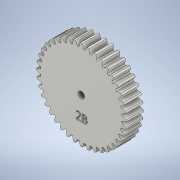
# Autodesk Inventor part: Spur Gear1
Saved by Autodesk Inventor 2021 (Build 250183000, 183)
## iProperties
CustomPartVersion: 1
Created: 2021-04-14
Part Number: Spur Gear1
Material: Steel
Document SubType Name: Modeling
Designer: Nabeel Azafer
Categories: <?xml version="1.0" encoding="UTF-16"?> <MemberInstance><Categories><FamilyTemplate><FamilyTemplateParameter ValueType="xs:double" Id="1" ObjectReferenceKey="da_z" ObjectType="kUserParameterObject"/><FamilyTemplateParameter ValueType="xs:double" Id="2" ObjectReferenceKey="da_b" ObjectType="kUserParameterObject"/><FamilyTemplateParameter ValueType="xs:double" Id="3" ObjectReferenceKey="da_beta" ObjectType="kUserParameterObject"/><FamilyTemplateParameter ValueType="xs:double" Id="4" ObjectReferenceKey="da_da" ObjectType="kUserParameterObject"/><FamilyTemplateParameter ValueType="xs:double" Id="5" ObjectReferenceKey="da_aw" ObjectType="kUserParameterObject"/><FamilyTemplateParameter ValueType="xs:string" Id="6" ObjectReferenceKey="EAIAABAAAACIAQAAAAAAAIAAAAAAAAAA" ObjectType="83910656" SubObjectId="SurfaceGeometry"/></FamilyTemplate><ParamToTemplateMap><ParamToTemplate CategoryParameter="//CategoryParameter[@InternalName='046C89C9-8512-4d59-83FE-43B91F4F132A']" TemplateParameter="1"/><ParamToTemplate CategoryParameter="//CategoryParameter[@InternalName='2552DF32-E462-4b46-AEBF-C6C7768E72AC']" TemplateParameter="2"/><ParamToTemplate CategoryParameter="//CategoryParameter[@InternalName='C9EE641D-15FC-4fae-A226-E94C4372FDD7']" TemplateParameter="3"/><ParamToTemplate><ParamToTemplate CategoryParameter="//CategoryParameter[@InternalName='00B6519A-459B-49c7-AD84-2E56D39A5744']" ConstantValue="0.000000"/></ParamToTemplate><ParamToTemplate><ParamToTemplate CategoryParameter="//CategoryParameter[@InternalName='04B31F0E-C7A6-4894-AA32-9629BEFACF47']" ConstantValue="0.800000"/></ParamToTemplate><ParamToTemplate><ParamToTemplate CategoryParameter="//CategoryParameter[@InternalName='43CBEC2E-7847-49e7-A936-2F7889FCB2D9']" ConstantValue="0.350000"/></ParamToTemplate><ParamToTemplate><ParamToTemplate CategoryParameter="//CategoryParameter[@InternalName='B1EFC894-105D-4ebd-86BF-FA20ED196853']" ConstantValue="0.500000"/></ParamToTemplate><ParamToTemplate><ParamToTemplate CategoryParameter="//CategoryParameter[@InternalName='51175063-3D10-4879-93E8-6246FE8B403D']" ConstantValue="2060000000.000000"/></ParamToTemplate><ParamToTemplate><ParamToTemplate CategoryParameter="//CategoryParameter[@InternalName='A3A52E27-4454-46a9-B0BD-C932399B70AF']" ConstantValue="0.300000"/></ParamToTemplate><ParamToTemplate><ParamToTemplate CategoryParameter="//CategoryParameter[@InternalName='91B76062-C214-41d9-B1B9-14D2AB99603D']" ConstantValue="0.100000"/></ParamToTemplate><ParamToTemplate><ParamToTemplate CategoryParameter="//CategoryParameter[@InternalName='374E806E-8B8A-4dda-A9AA-1039D6500AD2']" ConstantValue="10.000000"/></ParamToTemplate><ParamToTemplate><ParamToTemplate CategoryParameter="//CategoryParameter[@InternalName='2D373A89-B862-43d6-8D0B-0CBF12AB9F6C']" ConstantValue="0.349066"/></ParamToTemplate><ParamToTemplate CategoryParameter="//CategoryParameter[@InternalName='37777632-D6A2-4fac-9D53-DB8ACD95C989']" TemplateParameter="4"/><ParamToTemplate CategoryParameter="//CategoryParameter[@InternalName='FD1017F1-B727-4f7e-9707-0F86F1FF9423']" TemplateParameter="5"/><ParamToTemplate><ParamToTemplate CategoryParameter="//CategoryParameter[@InternalName='9E1B4470-B2D3-4ff1-B813-535BB4CDF51A']" ConstantValue="3520000.000000"/></ParamToTemplate><ParamToTemplate><ParamToTemplate CategoryParameter="//CategoryParameter[@InternalName='F8452263-BFF6-458c-9FB1-07C4B99E95CD']" ConstantValue="11400000.000000"/></ParamToTemplate><ParamToTemplate><ParamToTemplate CategoryParameter="//CategoryParameter[@InternalName='3E3BB259-FD49-497f-8171-6EBC954A3479']" ConstantValue="2.000000"/></ParamToTemplate><ParamToTemplate CategoryParameter="//CategoryParameter[@InternalName='27C3BAF2-7550-4e4b-AE2C-0DB134B7D9B7']" TemplateParameter="6"/></ParamToTemplateMap><Category DisplayName="Gear" InternalName="DC85795E-93AB-48d5-8EEE-5A27447B64BD" Mnemonic="Gear"><CategoryParameter DisplayName="z" InternalName="046C89C9-8512-4d59-83FE-43B91F4F132A" Mnemonic="z"/><CategoryParameter DisplayName="b" InternalName="2552DF32-E462-4b46-AEBF-C6C7768E72AC" Mnemonic="b"/><CategoryParameter DisplayName="||b|" InternalName="C9EE641D-15FC-4fae-A226-E94C4372FDD7" Mnemonic="beta"/><CategoryParameter DisplayName="x" InternalName="00B6519A-459B-49c7-AD84-2E56D39A5744" Mnemonic="x"/><CategoryParameter DisplayName="a*" InternalName="04B31F0E-C7A6-4894-AA32-9629BEFACF47" Mnemonic="a"/><CategoryParameter DisplayName="c*" InternalName="43CBEC2E-7847-49e7-A936-2F7889FCB2D9" Mnemonic="c"/><CategoryParameter DisplayName="r|.f|*" InternalName="B1EFC894-105D-4ebd-86BF-FA20ED196853" Mnemonic="rf"/><CategoryParameter DisplayName="E" InternalName="51175063-3D10-4879-93E8-6246FE8B403D" Mnemonic="E"/><CategoryParameter DisplayName="||m|" InternalName="A3A52E27-4454-46a9-B0BD-C932399B70AF" Mnemonic="mi"/><Category DisplayName="SpurGear" InternalName="26C5A22E-A91E-4dfd-A3B3-23CCAFAE1764" Mnemonic="SpurGear"><CategoryParameter DisplayName="m" InternalName="91B76062-C214-41d9-B1B9-14D2AB99603D" Mnemonic="m"/><CategoryParameter DisplayName="P" InternalName="374E806E-8B8A-4dda-A9AA-1039D6500AD2" Mnemonic="PP"/><CategoryParameter DisplayName="||a|" InternalName="2D373A89-B862-43d6-8D0B-0CBF12AB9F6C" Mnemonic="alpha"/><CategoryParameter DisplayName="d|.a|" InternalName="37777632-D6A2-4fac-9D53-DB8ACD95C989" Mnemonic="da"/><CategoryParameter DisplayName="a|.w|" InternalName="FD1017F1-B727-4f7e-9707-0F86F1FF9423" Mnemonic="aw"/><CategoryParameter DisplayName="||s||.Flim|" InternalName="9E1B4470-B2D3-4ff1-B813-535BB4CDF51A" Mnemonic="sFlim"/><CategoryParameter DisplayName="||s||.Hlim|" InternalName="F8452263-BFF6-458c-9FB1-07C4B99E95CD" Mnemonic="sHlim"/><CategoryParameter DisplayName="type" InternalName="3E3BB259-FD49-497f-8171-6EBC954A3479" Mnemonic="type"/><CategoryParameter DisplayName="PitchDiameter" InternalName="27C3BAF2-7550-4e4b-AE2C-0DB134B7D9B7" Mnemonic="IDS_PITCHDIAM"/></Category></Category></Categories></MemberInstance>
Density: 1 g/cm^3
Appearance: Steel
Author: Nabeel Azafer
Autodesk Inventor part; units mm, degrees
note: some values were not read from the file. Chosen so that the rebuilt part matches the saved one: direction of "Emboss1".
sketch "Sketch1" plane through (0, 0, 0) normal (0, 0, 1) x (1, 0, 0)
  circle A0 centre (0, 0) radius 20.7822
  dimension "d0" = 41.5644
  constraints: 1 centre point
  measures "d0" diameter of A0
extrude "Extrusion1" add sketch "Sketch1" along normal blind 8
ref_plane "Work Plane2" through (0, 0, 4) normal (0, 0, 1) x (1, 0, 0)
sketch "Sketch2" plane through (0, 0, 0) normal (0, 0, -1) x (-1, 0, 0)
  circle A0 centre (0, 0) radius 20.7822 projected
  circle A1 centre (0, 0) radius 20
  dimension "d3" = 40
  constraints: 1 centre point, 1 coincident
  measures "d3" diameter of A1
surface extrude "Pitch Diameter" sketch "Sketch2" against normal through all shown no curves A1
ref_plane "Work Plane8" through (0, 0, 0) normal (0.9969173, 0.0784591, 0) x (0, 0, 1)
ref_plane "Work Plane9" through (0, 0, 0) normal (1, 0, 0) x (0, 1, 0)
spur gear teeth "Spur Gear" teeth 40 pitch diameter 40 tip diameter 41.5644 root diameter 37.7 face width 8 start plane through (0, 0, 0) normal (0, 0, -1) x (-1, 0, 0)
sketch "Sketch3" plane through (0, 0, 8) normal (0, 0, 1) x (1, 0, 0)
  point P0 (0, 0)
sketch "Sketch4" plane through (0, 0, 8) normal (0, 0, 1) x (1, 0, 0)
  circle A0 centre (0, 0) radius 1.5
  dimension "d49" = 3
  constraints: 1 centre point, 1 coincident
  measures "d49" diameter of A0
hole "Hole1" at (0, 0, 8) direction (0, 0, -1) diameter 3 end through all
sketch "Sketch5" plane through (0, 0, 8) normal (0, 0, 1) x (1, 0, 0)
  line L0 (-2.5799, -7.1656) -> (7.9916, -7.1656) construction
  line L1 (7.9916, -7.1656) -> (7.9916, -18.7281) construction
  line L2 (7.9916, -18.7281) -> (-2.5799, -18.7281) construction
  line L3 (-2.5799, -18.7281) -> (-2.5799, -7.1656) construction
  line L4 (-0.1662, -10.7393) -> (-2.3246, -10.7393)
  line L5 (-2.3246, -10.7393) -> (-2.3246, -10.243)
  spline S0 degree 2 poles (-2.3246, -10.243) (-2.092, -10.0246) (-1.6779, -9.619) (-1.4794, -9.4006) knots 0 0 0 1 2 2 2
  spline S1 degree 2 poles (-1.4794, -9.4006) (-1.0795, -8.961) (-0.7873, -8.4334) (-0.7873, -8.1526) knots 0 0 0 1 2 2 2
  spline S2 degree 2 poles (-0.7873, -8.1526) (-0.7873, -8.0051) (-0.8781, -7.7839) (-0.9603, -7.713) knots 0 0 0 1 2 2 2
  spline S3 degree 2 poles (-0.9603, -7.713) (-1.0426, -7.6421) (-1.2581, -7.5712) (-1.3886, -7.5712) knots 0 0 0 1 2 2 2
  spline S4 degree 2 poles (-1.3886, -7.5712) (-1.5134, -7.5712) (-1.7687, -7.6336) (-1.885, -7.6818) knots 0 0 0 1 2 2 2
  spline S5 degree 2 poles (-1.885, -7.6818) (-1.9842, -7.7215) (-2.1686, -7.835) (-2.2253, -7.8747) knots 0 0 0 1 2 2 2
  line L6 (-2.2253, -7.8747) -> (-2.2509, -7.8747)
  line L7 (-2.2509, -7.8747) -> (-2.2509, -7.3755)
  spline S6 degree 2 poles (-2.2509, -7.3755) (-2.1062, -7.3046) (-1.5872, -7.1656) (-1.3546, -7.1656) knots 0 0 0 1 2 2 2
  spline S7 degree 2 poles (-1.3546, -7.1656) (-0.8639, -7.1656) (-0.3108, -7.6846) (-0.3108, -8.1271) knots 0 0 0 1 2 2 2
  spline S8 degree 2 poles (-0.3108, -8.1271) (-0.3108, -8.3342) (-0.4073, -8.6802) (-0.4923, -8.8277) knots 0 0 0 1 2 2 2
  spline S9 degree 2 poles (-0.4923, -8.8277) (-0.5774, -8.9808) (-0.8242, -9.2815) (-0.9603, -9.4261) knots 0 0 0 1 2 2 2
  spline S10 degree 2 poles (-0.9603, -9.4261) (-1.1816, -9.6672) (-1.7233, -10.1834) (-1.885, -10.3338) knots 0 0 0 1 2 2 2
  line L8 (-1.885, -10.3338) -> (-0.1662, -10.3338)
  line L9 (-0.1662, -10.3338) -> (-0.1662, -10.7393)
  spline S11 degree 2 poles (2.7751, -9.6644) (2.7751, -9.9253) (2.5765, -10.3252) (2.412, -10.4557) knots 0 0 0 1 2 2 2
  spline S12 degree 2 poles (2.412, -10.4557) (2.2135, -10.6089) (1.7625, -10.7393) (1.4051, -10.7393) knots 0 0 0 1 2 2 2
  line L10 (1.4051, -10.7393) -> (0.4011, -10.7393)
  line L11 (0.4011, -10.7393) -> (0.4011, -7.2393)
  line L12 (0.4011, -7.2393) -> (1.3286, -7.2393)
  spline S13 degree 2 poles (1.3286, -7.2393) (1.703, -7.2393) (2.0773, -7.2876) (2.2475, -7.3812) knots 0 0 0 1 2 2 2
  spline S14 degree 2 poles (2.2475, -7.3812) (2.4376, -7.4804) (2.6106, -7.8066) (2.6106, -8.0278) knots 0 0 0 1 2 2 2
  spline S15 degree 2 poles (2.6106, -8.0278) (2.6106, -8.2746) (2.3496, -8.666) (2.1199, -8.7766) knots 0 0 0 1 2 2 2
  line L13 (2.1199, -8.7766) -> (2.1199, -8.7936)
  spline S16 degree 2 poles (2.1199, -8.7936) (2.4319, -8.8787) (2.7751, -9.3297) (2.7751, -9.6644) knots 0 0 0 1 2 2 2
  spline S17 degree 2 poles (2.2901, -9.6842) (2.2901, -9.4857) (2.1766, -9.2304) (2.0064, -9.1397) knots 0 0 0 1 2 2 2
  spline S18 degree 2 poles (2.0064, -9.1397) (1.8958, -9.0829) (1.6349, -9.0489) (1.3938, -9.0489) knots 0 0 0 1 2 2 2
  line L14 (1.3938, -9.0489) -> (0.8662, -9.0489)
  line L15 (0.8662, -9.0489) -> (0.8662, -10.3423)
  line L16 (0.8662, -10.3423) -> (1.2435, -10.3423)
  spline S19 degree 2 poles (1.2435, -10.3423) (1.5498, -10.3423) (1.9015, -10.2855) (2.0376, -10.1948) knots 0 0 0 1 2 2 2
  spline S20 degree 2 poles (2.0376, -10.1948) (2.1681, -10.1012) (2.2901, -9.8686) (2.2901, -9.6842) knots 0 0 0 1 2 2 2
  spline S21 degree 2 poles (2.1256, -8.0931) (2.1256, -7.9683) (2.0405, -7.7811) (1.9469, -7.7272) knots 0 0 0 1 2 2 2
  spline S22 degree 2 poles (1.9469, -7.7272) (1.8334, -7.6648) (1.5583, -7.6364) (1.3115, -7.6364) knots 0 0 0 1 2 2 2
  line L17 (1.3115, -7.6364) -> (0.8662, -7.6364)
  line L18 (0.8662, -7.6364) -> (0.8662, -8.6603)
  line L19 (0.8662, -8.6603) -> (1.3938, -8.6603)
  spline S23 degree 2 poles (1.3938, -8.6603) (1.6122, -8.6603) (1.8192, -8.6149) (1.9299, -8.544) knots 0 0 0 1 2 2 2
  spline S24 degree 2 poles (1.9299, -8.544) (2.0376, -8.476) (2.1256, -8.2576) (2.1256, -8.0931) knots 0 0 0 1 2 2 2
  point P0 (0, 0)
  constraints: 2 other
emboss "Emboss1" sketch "Sketch5" operation cut depth 1 direction (0, 0, -1)
equation "\"d0\" = da_da"
equation "\"d1\" = da_b"
equation "\"d3\" = da_d"
equation "\"d16\" = da_aw"
equation "\"d43\" = da_aw"
equation "\"d46\" = da_aw"
equation "\"da_da\" = 41.564361"
equation "\"da_b\" = 8"
equation "\"da_d\" = 40"
equation "\"da_aw\" = 25.351695"
body "Solid1"
body "Srf1"
